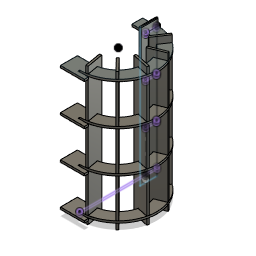
bending rig v1 (Autodesk Fusion 360 design; units mm, degrees)
Autodesk Fusion 360 part; units mm, degrees
sketch "Sketch1" plane through (0, 0, 0) normal (0, 1, 0) x (1, 0, 0)
  line L0 (0, 0) -> (0, 63.9553)
  line L1 (0, 0) -> (0, -73.7364)
  arc A0 (0, -58.735) -> (0, 58.735) centre (0, 0) ccw
  arc A1 (0, -56.735) -> (0, 56.735) centre (0, 0) ccw
  dimension "d1" = 117.47
  constraint coincident L0.start L1.start
  constraint vertical L0
  constraint parallel L0 L1
  constraint coincident L0 A0.end
  constraint coincident L1 A0.start
  constraint coincident L0 A1.end
  constraint coincident L1 A1.start
  measures "d1" diameter of A0
extrude "Extrude1" add sketch "Sketch1" along normal blind 250 contours L0 L1 A0 A1 makes body 1
ref_plane "WorkPlane1" through (29.3675, 210, 0) normal (0, 1, 0) x (1, 0, 0)
sketch "Sketch2" plane through (29.3675, 210, 0) normal (0, 1, 0) x (1, 0, 0)
  arc A0 (-29.3675, -58.735) -> (-29.3675, 58.735) centre (-29.3675, 0) ccw
  line L0 (-29.3675, 58.735) -> (-29.3675, 56.735)
  arc A1 (-29.3675, -56.735) -> (-29.3675, 56.735) centre (-29.3675, 0) ccw
  line L1 (-29.3675, -56.735) -> (-29.3675, -58.735)
  arc A2 (-29.3675, -40.0209) -> (-29.3675, 40.0209) centre (-29.3675, 0) ccw
  line L2 (-29.3675, -40.0209) -> (-49.3675, -40.0209)
  line L3 (-49.3675, -40.0209) -> (-49.3675, -65.0209)
  line L4 (-49.3675, -65.0209) -> (-29.3675, -65.0209)
  line L5 (-29.3675, -59.0471) -> (-29.3675, -56.735)
  line L6 (-29.3675, 40.0209) -> (-49.3675, 40.0209)
  line L7 (-49.3675, 40.0209) -> (-49.3675, 55.6991)
  line L8 (-49.3675, 55.6991) -> (-29.3675, 55.6991)
  line L9 (-29.3675, 56.735) -> (-29.3675, 55.6991)
  line L10 (-29.3675, -65.0209) -> (-14.1787, -65.0209)
  line L11 (-14.1787, -65.0209) -> (-14.1787, -59.0471)
  line L12 (-14.1787, -59.0471) -> (-29.3675, -59.0471)
  dimension "d7" = 20
  dimension "d8" = 25
  dimension "d9" = 20
  constraint coincident L0.end A1.end
  constraint concentric A1 A2
  constraint coincident A2.end L9
  constraint coincident A2.start L9
  constraint horizontal L2
  constraint vertical L3
  constraint horizontal L4
  constraint vertical L5
  constraint horizontal L6
  constraint vertical L7
  constraint horizontal L8
  constraint horizontal L10
  constraint vertical L11
  constraint horizontal L12
  measures "d7" distance of A2.start L2.end
  measures "d8" distance of A2.start L4.end
  measures "d9" distance of A2.end L6.end
extrude "Extrude2" add sketch "Sketch2" along normal blind 3 separate body contours A1 L1 A2 L2 L3 L4 L5 L6 L7 L8 L9 L10 L11 L12 makes body 2
pattern_linear "R-Pattern1" count 4 spacing 60 along (0, -1, 0) of bodies 2 makes body 3 at (-13.3333, 150, 53.9256) makes body 4 at (-13.3333, 90, 53.9256) makes body 5 at (-13.3333, 30, 53.9256)
sketch "Sketch3" plane through (0, 0, 0) normal (-1, 0, 0) x (0, 0, 1)
  line L0 (-56.735, 210) -> (-55.6991, 210)
  line L1 (-55.6991, 210) -> (-55.6991, 213)
  line L2 (-55.6991, 213) -> (-56.735, 213)
  line L3 (-56.735, 213) -> (-56.735, 210)
  line L4 (-56.735, 213) -> (-56.735, 223) construction
  line L5 (-56.735, 223) -> (-31.9786, 223)
  line L6 (-31.9786, 223) -> (-31.9786, 21.4848)
  line L7 (-31.9786, 21.4848) -> (-56.735, 21.4848)
  line L8 (-56.735, 21.4848) -> (-56.735, 223)
  line L9 (-55.6991, 210) -> (-40.0209, 210)
  line L10 (-40.0209, 210) -> (-40.0209, 213)
  line L11 (-40.0209, 213) -> (-55.6991, 213)
  line L12 (-55.6991, 213) -> (-55.6991, 210)
  line L13 (-55.6991, 150) -> (-40.0209, 150)
  line L14 (-40.0209, 150) -> (-40.0209, 153)
  line L15 (-40.0209, 153) -> (-55.6991, 153)
  line L16 (-55.6991, 153) -> (-55.6991, 150)
  line L17 (-56.735, 150) -> (-55.6991, 150)
  line L18 (-55.6991, 150) -> (-55.6991, 153)
  line L19 (-55.6991, 153) -> (-56.735, 153)
  line L20 (-56.735, 153) -> (-56.735, 150)
  line L21 (-55.6991, 90) -> (-40.0209, 90)
  line L22 (-40.0209, 90) -> (-40.0209, 93)
  line L23 (-40.0209, 93) -> (-55.6991, 93)
  line L24 (-55.6991, 93) -> (-55.6991, 90)
  line L25 (-56.735, 90) -> (-55.6991, 90)
  line L26 (-55.6991, 90) -> (-55.6991, 93)
  line L27 (-55.6991, 93) -> (-56.735, 93)
  line L28 (-56.735, 93) -> (-56.735, 90)
  line L29 (56.735, 30) -> (-56.735, 30)
  line L30 (-56.735, 30) -> (-56.735, 33)
  line L31 (56.735, 33) -> (-56.735, 33)
  line L32 (56.735, 33) -> (56.735, 30)
  line L33 (-40.0209, 93) -> (-40.0209, 25.2601) construction
  line L34 (-40.0209, 33) -> (-40.0209, 30)
  dimension "d16" = 10
  constraint coincident L2.end L3.start
  constraint perpendicular L2 L4
  constraint horizontal L5
  constraint vertical L6
  constraint horizontal L7
  constraint vertical L8
  constraint coincident L22.end L23.start
  constraint perpendicular L7 L33
  constraint coincident L33 L34.start
  constraint coincident L31 L34.start
  constraint coincident L33 L34.end
  constraint coincident L29 L34.end
  measures "d16" distance of L2.end L4.end
extrude "Extrude3" add sketch "Sketch3" along normal mid plane 3 separate body contours L0 L2 L5 L6 L8 L9 L10 L11 L13 L14 L15 L17 L19 L21 L22 L23 L25 L27 L31 | L6 L29 L31 L34 | L6 L7 L8 L29 | L8 L29 L30 L31 L34 makes body 6
sketch "Sketch4" plane through (0, 213, 0) normal (0, 1, 0) x (-1, 0, 0)
  line L0 (0, 40.0209) -> (20, 40.0209)
  line L1 (20, 40.0209) -> (20, 65.0209)
  line L2 (20, 65.0209) -> (-15.1888, 65.0209)
  line L3 (-15.1888, 65.0209) -> (-15.1888, 59.0471)
  line L4 (-15.1888, 59.0471) -> (0, 59.0471)
  line L5 (0, 59.0471) -> (0, 56.735)
  arc A0 (0, 56.735) -> (0, -56.735) centre (0, 0) ccw
  line L6 (0, -56.735) -> (0, -55.6991)
  line L7 (0, -55.6991) -> (20, -55.6991)
  line L8 (20, -55.6991) -> (20, -40.0209)
  line L9 (20, -40.0209) -> (0, -40.0209)
  arc A1 (0, 40.0209) -> (0, -40.0209) centre (0, 0) ccw
  constraint coincident A0.centre A1.centre
extrude "Extrude4" cut sketch "Sketch3" along normal blind 25 contours L8 L29 L30 L31 L34 bodies 6
extrude "Extrude5" cut sketch "Sketch3" against normal blind 18 contours L8 L29 L30 L31 L34 bodies 6
delete_body "RemoveBody1" bodies 1
pattern_circular "C-Pattern1" count 6 over 170 about axis through (0, 1.75, 0) along (0, -1, 0) of bodies 6 makes body 7 at (29.8539, 131, -41.5778) makes body 8 at (48, 71, -17.7755) makes body 9 at (44.9078, 131, 8.0119) makes body 10 at (30.592, 71, 33.8383) makes body 11 at (7.4073, 71, 50.6468)
named bodies: "Ring 1", "Ring 2", "Ring 3", "Rib 1", "Ring 4", "Rib 1 (1)", "Rib 1 (2)", "Rib 1 (3)", "Rib 1 (4)", "Rib 1 (5)"
